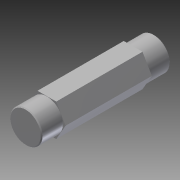
# Autodesk Inventor part: DBK_SmallHexShaft_am-0152
Saved by Autodesk Inventor 2015 (Build 190159000, 159)
## iProperties
Category: Drive Base Kit
Company: Autodesk Inc.
Created: 2012-12-19
Part Number: DBK_SmallHexShaft_am-0152
Material: Steel
Document SubType Name: Modeling
Designer: Autodesk Inc.
Density: 7.83431 g/cm^3
Catalog Web Link: http://www.andymark.com/product-p/am-0152.htm
Vendor: AndyMark Inc.
Mass: 22.6796 g
Surface Area: 13.656 cm^2
Volume: 2.89491 cm^3
Appearance: Steel
Author: Autodesk Inc.
Autodesk Inventor part; units mm, degrees
ref_plane "YZ Plane" through (0, 0, 0) normal (1, 0, 0) x (0, 1, 0)
ref_plane "XZ Plane" through (0, 0, 0) normal (0, 1, 0) x (-1, 0, 0)
sketch "Sketch1" plane through (0, 0, 0) normal (0, 0, 1) x (1, 0, 0)
  line L0 (2.7496, 4.7625) -> (5.4993, 0)
  line L1 (5.4993, 0) -> (2.7496, -4.7625)
  line L2 (2.7496, -4.7625) -> (-2.7496, -4.7625)
  line L3 (-2.7496, -4.7625) -> (-5.4993, 0)
  line L4 (-5.4993, 0) -> (-2.7496, 4.7625)
  line L5 (-2.7496, 4.7625) -> (2.7496, 4.7625)
  point P0 (0, 0)
  point P1 (0, 0)
  dimension "d0" = 9.525
  constraints: 12 end point, 1 coincident, 1 horizontal, 13 other
  measures "d0" distance between parallel lines of L2 L5
extrude "Extrusion1" add sketch "Sketch1" against normal blind 38.1
sketch "Sketch2" plane through (0, 0, 0) normal (0, 0, 1) x (1, 0, 0)
  line L0 (2.7496, 4.7625) -> (5.4993, 0) projected
  line L1 (-2.7496, 4.7625) -> (2.7496, 4.7625) projected
  line L2 (-5.4993, 0) -> (-2.7496, 4.7625) projected
  line L3 (-2.7496, -4.7625) -> (-5.4993, 0) projected
  line L4 (2.7496, -4.7625) -> (-2.7496, -4.7625) projected
  line L5 (5.4993, 0) -> (2.7496, -4.7625) projected
  circle A0 centre (0, 0) radius 4.7625
  dimension "d3" = 9.525
  constraints: 1 centre point, 1 coincident
  measures "d3" diameter of A0
extrude "Extrusion2" cut sketch "Sketch2" against normal blind 6.2865 contours L0 A0 L1 | L0 L5 A0 | A0 L2 L1 | A0 L3 L2 | L5 L4 A0 | A0 L4 L3
ref_plane "Work Plane1" through (0, 0, -19.05) normal (0, 0, 1) x (1, 0, 0)
mirror "Mirror1" about plane through (0, 0, -19.05) normal (0, 0, 1) of "Extrusion2"
sketch "Sketch3" plane through (2.7496, -4.7625, -31.8135) normal (0, 0, -1) x (-1, 0, 0)
  line L0 (5.5213, 9.5631) -> (8.2929, 4.7625)
  line L1 (8.2929, 4.7625) -> (5.5213, -0.0381)
  line L2 (5.5213, -0.0381) -> (-0.022, -0.0381)
  line L3 (-0.022, -0.0381) -> (-2.7936, 4.7625)
  line L4 (-2.7936, 4.7625) -> (-0.022, 9.5631)
  line L5 (-0.022, 9.5631) -> (5.5213, 9.5631)
  line L6 (0, 9.525) -> (5.4993, 9.525) projected
  point P0 (2.7496, 4.7625)
  point P1 (2.7496, 4.7625)
  dimension "d11" = 9.6012
  constraints: 12 end point, 1 coincident, 1 parallel, 13 other
  measures "d11" distance between parallel lines of L2 L5
extrude "Extrusion3" add sketch "Sketch3" against normal blind 44.45
sketch "Sketch5" plane through (2.7496, -4.7625, 12.6365) normal (0, 0, 1) x (1, 0, 0)
  circle A0 centre (-2.7496, 4.7625) radius 4.7625
  dimension "d15" = 9.525
  constraints: 1 centre point, 1 coincident
  measures "d15" diameter of A0
extrude "Extrusion4" add sketch "Sketch5" along normal blind 6.2992
chamfer "Chamfer1" distance 0.254 angle 45 2 edges at (-4.1244, -2.3812, -38.1) (-4.7625, 0, 18.9357)
body "Solid1"
